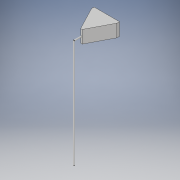
# Autodesk Inventor part: Part2
Saved by Autodesk Inventor 2019 (Build 230136000, 136)
## iProperties
Created: 2020-02-12
Part Number: Part2
Material: Generic
Document SubType Name: Modeling
Designer: ASUS
Density: 1 g/cm^3
Appearance: Default
Author: ASUS
Autodesk Inventor part; units mm, degrees
ref_plane "YZ Plane" through (0, 0, 0) normal (1, 0, 0) x (0, 1, 0)
ref_plane "XZ Plane" through (0, 0, 0) normal (0, 1, 0) x (-1, 0, 0)
ref_plane "XY Plane" through (0, 0, 0) normal (0, 0, 1) x (1, 0, 0)
sketch "Sketch1" plane through (0, 0, 0) normal (0, 1, 0) x (-1, 0, 0)
  line L0 (0, 0) -> (100, 0)
  line L1 (100, 0) -> (100, 100)
  line L2 (100, 100) -> (0, 100)
  line L3 (0, 100) -> (0, 0)
  dimension "d0" = 100
  dimension "d1" = 100
  constraints: 8 end point, 2 parallel, 1 horizontal, 1 perpendicular
  measures "d0" distance of L2.end L1.end
  measures "d1" distance of L1.end L0.end
extrude "Extrusion1" add sketch "Sketch1" along normal blind 50
chamfer "Chamfer1" distance 47 distance2 90 1 edges at (0, 25, 100) measured on face at (-0.5, 25, 100)
chamfer "Chamfer2" distance 90 distance2 47 1 edges at (-100, 25, 100) measured on face at (-100, 25, 99.5)
sketch "Sketch2" plane through (-47, 0, 100) normal (0, 0, 1) x (1, 0, 0)
  circle A0 centre (-2.7639, 25) radius 2.5
  point P0 (47, 0)
  dimension "d10" = 5
  constraints: 1 centre point
  measures "d10" diameter of A0
extrude "Extrusion2" add sketch "Sketch2" along normal blind 30
sketch "Sketch3" plane through (0, 0, 0) normal (0, 1, 0) x (-1, 0, 0)
  line L0 (52.2639, 130) -> (47.2639, 130) projected
  circle A0 centre (49.7639, 130) radius 2.5
  point P0 (0, 0)
  constraints: 1 horizontal alignment, 1 midpoint, 2 other
extrude "Extrusion3" add sketch "Sketch3" along normal blind 27 and the other way blind 400
shell "Shell1" thickness 1 removed faces 1 at (-33.3333, 16.6667, 0)
body "Solid1"
